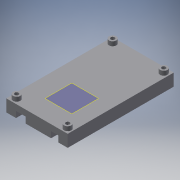
# Autodesk Inventor part: J120_Mount
Saved by Autodesk Inventor 2018 (Build 220112000, 112)
## iProperties
Created: 2017-04-11
Part Number: J120_Mount
Material: 一般
Document SubType Name: Modeling
Designer: g45k
Mass: 41.586 g
Surface Area: 153.784 cm^2
Volume: 41.586 cm^3
Density: 1 g/cm^3
Appearance: 既定
Author: g45k
Autodesk Inventor part; units mm, degrees
ref_plane "YZ Plane" through (0, 0, 0) normal (1, 0, 0) x (0, 1, 0)
ref_plane "XZ Plane" through (0, 0, 0) normal (0, 1, 0) x (-1, 0, 0)
ref_plane "XY Plane" through (0, 0, 0) normal (0, 0, 1) x (1, 0, 0)
sketch "スケッチ2" plane through (0, 0, 0) normal (0, 0, 1) x (1, 0, 0)
  line L0 (-28, 61.5) -> (-28, 48.6) construction
  line L1 (-28.1, 61.4) -> (22.5, 61.4)
  line L2 (22.5, 61.4) -> (22.5, -25.9)
  line L3 (22.5, -25.9) -> (-28.1, -25.9)
  line L4 (-28.1, -25.9) -> (-28.1, 61.4)
  line L5 (28, 48.6) -> (28, 61.5) construction
  circle A0 centre (-23.5, -21.9) radius 1.6 construction
  circle A1 centre (-23.5, 57.1) radius 1.6 construction
  circle A2 centre (18.5, 57.1) radius 1.6 construction
  circle A3 centre (18.5, -21.9) radius 1.6 construction
  circle A4 centre (18.5, 57.1) radius 1.6
  circle A5 centre (-23.5, 57.1) radius 1.6
  circle A6 centre (18.5, -21.9) radius 1.6
  circle A7 centre (-23.5, -21.9) radius 1.6
  line L6 (28, 61.5) -> (-28, 61.5) construction
  point P0 (0, 0)
extrude "押し出し1" add sketch "スケッチ2" along normal blind 10
sketch "スケッチ3" plane through (0, 0, 0) normal (0, 0, -1) x (-1, 0, 0)
  circle A0 centre (3.1, 21.4) radius 21.1
  line L0 (28.1, 61.4) -> (-22.5, 61.4) construction
  line L1 (28.1, -25.9) -> (28.1, 61.4) construction
  dimension "d7" = 42.2
  dimension "d107" = 40
  dimension "d108" = 25
  constraints: 1 centre point
  measures "d7" diameter of A0
  measures "d107" distance from line of L0 A0.centre
  measures "d108" distance from line of L1 A0.centre
extrude "押し出し2" cut sketch "スケッチ3" against normal blind 6
sketch "スケッチ4" plane through (-3.1, 21.4, 6) normal (0, 0, -1) x (-1, 0, 0)
  circle A0 centre (4.5753, -17.0753) radius 3
  circle A1 centre (-17.0753, -4.5753) radius 3
  circle A2 centre (17.0753, 4.5753) radius 3
  circle A3 centre (-4.5753, 17.0753) radius 3
  line L0 (4.5753, -17.0753) -> (-17.0753, -4.5753) construction
  line L1 (-17.0753, -4.5753) -> (-4.5753, 17.0753) construction
  line L2 (-4.5753, 17.0753) -> (17.0753, 4.5753) construction
  line L3 (17.0753, 4.5753) -> (4.5753, -17.0753) construction
  line L4 (27.9, -40.8029) -> (27.9, 46.5471) construction
  line L5 (-4.5753, 17.0753) -> (4.5753, -17.0753) construction
  line L6 (-17.0753, -4.5753) -> (17.0753, 4.5753) construction
  circle A4 centre (0, 0) radius 21.1 construction
  point P0 (0, 0)
  dimension "d89" = 3.5
  dimension "d22" = 6
  dimension "d23" = 25
  dimension "d24" = 25
  dimension "d25" = 30
  constraints: 14 end point, 4 centre point, 3 equal radius, 3 perpendicular, 2 midpoint, 1 coincident
  measures "d22" diameter of A0
  measures "d23" distance of L0.end L1.end
  measures "d24" distance of L1.end L2.end
  measures "d25" angle of L3 L4
extrude "押し出し3" add sketch "スケッチ4" along normal blind 1
sketch "スケッチ6" plane through (-7.6753, 4.3247, 5) normal (0, 0, -1) x (-1, 0, 0)
  circle A0 centre (0, 0) radius 3 construction
  circle A1 centre (-21.6506, 12.5) radius 3 construction
  circle A2 centre (-9.1506, 34.1506) radius 3 construction
  circle A3 centre (-4.5753, 17.0753) radius 21.1 construction
  circle A4 centre (0, 0) radius 1.45
  circle A5 centre (-9.1506, 34.1506) radius 1.45
  circle A6 centre (-21.6506, 12.5) radius 1.45
  circle A7 centre (12.5, 21.6506) radius 3 construction
  circle A8 centre (12.5, 21.6506) radius 1.45
  dimension "d15" = 2.9
  constraints: 8 centre point, 4 coincident, 3 equal radius
  measures "d15" diameter of A4
extrude "押し出し5" add sketch "スケッチ6" along normal blind 1
sketch "スケッチ8" plane through (0, 0, 0) normal (0, 0, -1) x (-1, 0, 0)
  circle A0 centre (3.1, 21.4) radius 21.1 construction
  line L0 (20, 8.7667) -> (20, -25.9)
  line L1 (-22.5, -25.9) -> (28.1, -25.9) projected
  line L2 (20, -25.9) -> (12, -25.9)
  line L3 (28.1, -25.9) -> (-22.5, -25.9) projected
  line L4 (12, -25.9) -> (12, 2.2689)
  circle A1 centre (23.5, -21.9) radius 1.6 construction
  circle A2 centre (3.1, 21.4) radius 21.1 construction
  line L5 (23, 28.4143) -> (23, 43.0571)
  line L6 (6, 42.2998) -> (6, 43.0571)
  arc A3 (23, 43.0571) -> (6, 43.0571) centre (14.5, 43.0571) ccw
  arc A4 (23, 28.4143) -> (6, 42.2998) centre (3.1, 21.4) ccw
  arc A5 (12, 2.2689) -> (20, 8.7667) centre (3.1, 21.4) ccw
  point P0 (0, 0)
  dimension "d114" = 8
  dimension "d115" = 3.5
  dimension "d129" = 3
  dimension "d130" = 8.5
  constraints: 12 point on circle, 10 end point, 4 vertical, 3 centre point, 2 coincident, 2 point on line, 2 tangent
  measures "d114" distance between parallel lines of L0 L4
  measures "d115" distance from line of L0 A1.centre
  measures "d129" distance between parallel lines of L5 L0
  measures "d130" radius of A3
extrude "押し出し7" cut sketch "スケッチ8" against normal blind 6
ref_plane "作業平面1" through (-7.6753, 4.3247, 3.75) normal (0, 0, -1) x (-1, 0, 0)
sketch "スケッチ10" plane through (0, 0, 0) normal (0, 0, -1) x (-1, 0, 0)
  arc A0 (6, 42.2998) -> (12, 2.2689) centre (3.1, 21.4) ccw projected
  line L0 (-11.4796, 6.1473) -> (-17.6642, -4.5647)
  line L1 (-17.6642, -4.5647) -> (-17.6642, -12.3883)
  line L2 (-22.5, -25.9) -> (28.1, -25.9) projected
  line L3 (-14.7881, -25.9) -> (-8.7881, -25.9)
  line L4 (-8.7881, -25.9) -> (-8.7881, -9.1908)
  line L5 (-8.7881, -9.1908) -> (-2.8194, 1.1473)
  line L6 (3.1, 21.4) -> (-11.9, -4.5808) construction
  line L7 (3.1, 21.4) -> (33.1, 21.4) construction
  line L8 (-14.7881, -25.9) -> (-14.7881, -16.3883)
  line L9 (-14.7881, -16.3883) -> (-17.6642, -12.3883)
  point P0 (20, 8.7667)
  point P1 (12, -25.9)
  point P2 (23, 28.4143)
  dimension "d111" = 30
  dimension "d112" = 120
  dimension "d117" = 10
  dimension "d118" = 6
  dimension "d119" = 4
  constraints: 18 end point, 3 vertical, 2 parallel, 2 point on circle, 1 equal length, 1 horizontal, 1 point on line, 1 other
  measures "d111" distance of L6.start L6.end
  measures "d112" angle of L6 L7
  measures "d117" distance between parallel lines of L5 L0
  measures "d118" distance between parallel lines of L4 L8
  measures "d119" vertical distance of L1.end L8.end
extrude "押し出し9" cut sketch "スケッチ10" against normal blind 6
ref_plane "作業平面2" through (0, 0, 5) normal (0, 0, -1) x (-1, 0, 0)
ref_plane "作業平面3" through (0, 0, 7) normal (0, 0, 1) x (1, 0, 0)
ref_plane "作業平面4" through (0, 0, 11) normal (0, 0, -1) x (-1, 0, 0)
sketch "スケッチ18" plane through (0, 0, 10) normal (0, 0, 1) x (1, 0, 0)
  circle A0 centre (18.5, -21.9) radius 1.6 projected
  circle A1 centre (18.5, -21.9) radius 3
  circle A2 centre (-23.5, -21.9) radius 1.6 projected
  circle A3 centre (-23.5, -21.9) radius 3
  circle A4 centre (18.5, 57.1) radius 1.6 projected
  circle A5 centre (18.5, 57.1) radius 3
  circle A6 centre (-23.5, 57.1) radius 1.6 projected
  circle A7 centre (-23.5, 57.1) radius 3
  point P0 (0, 0)
  dimension "d85" = 6
  dimension "d86" = 6
  dimension "d87" = 6
  dimension "d110" = 6
  constraints: 4 centre point, 4 coincident
  measures "d85" diameter of A1
  measures "d86" diameter of A3
  measures "d87" diameter of A5
  measures "d110" diameter of A7
extrude "押し出し17" add sketch "スケッチ18" along normal blind 3.5
sketch "スケッチ21" plane through (-7.6753, 4.3247, 3.75) normal (0, 0, -1) x (-1, 0, 0)
  arc A0 (-1.6753, 37.9751) -> (4.3247, -2.0558) centre (-4.5753, 17.0753) ccw construction
  line L0 (-4.5753, 17.0753) -> (-22.8485, 27.6253) construction
  line L1 (-4.5753, 17.0753) -> (16.5247, 17.0753) construction
  circle A1 centre (-4.5753, 17.0753) radius 21.1
  circle A2 centre (-4.5753, 17.0753) radius 19.6
  line L2 (-22.2496, 25.5475) -> (-23.5522, 26.2996)
  arc A3 (-1.6753, 37.9751) -> (-19.155, 1.8226) centre (-4.5753, 17.0753) ccw projected
  line L3 (-20.7496, 28.1456) -> (-22.0522, 28.8977)
  line L4 (12.9016, 5.253) -> (11.599, 6.005)
  arc A4 (-1.6753, 37.9751) -> (4.3247, -2.0558) centre (-4.5753, 17.0753) ccw projected
  line L5 (14.4016, 7.851) -> (13.099, 8.6031)
  point P0 (-7.6753, -4.3247)
  point P1 (15.3247, 24.0896)
  point P2 (12.3247, 4.442)
  point P3 (-10.4947, -3.1774)
  dimension "d120" = 150
  dimension "d121" = 1.5
  dimension "d122" = 3
  dimension "d123" = 3
  constraints: 12 end point, 12 point on circle, 2 centre point, 2 coincident, 2 parallel, 1 concentric, 1 equal length, 1 horizontal, 2 other
  measures "d120" angle of L1 L0
  measures "d121" radial gap between concentric circles of A2 A1
  measures "d122" distance between parallel lines of L2 L3
  measures "d123" distance between parallel lines of L5 L4
extrude "押し出し19" add sketch "スケッチ21" along normal blind 2 contours A1 L4 A2 L5 | L3 A2 L2 A1
chamfer "面取り5" distance 1.4 angle 45 2 edges at (-20.0741, 11.6, 1.75) (13.8741, 31.2, 1.75)
